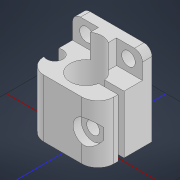
# Autodesk Inventor part: Vinda_Mount_v2
Saved by Autodesk Inventor 2022 (Build 260153000, 153)
## iProperties
Created: 2022-02-14
Part Number: Vinda_Mount_v2
Material: Stahl
Document SubType Name: Modeling
Designer: sleib
Density: 7.85 g/cm^3
Appearance: Vorgabe
Sending System: Autodesk Translation Framework v10.10.0.1391
Preprocessor: ST-DEVELOPER v18.1
Title: C:/Users/sleib/Projekte/Voron-2/STLs/VORON2.4/Gantry/X_Axis/X_Carriage/Vinda_Mount v4.step
Autodesk Inventor part; units mm, degrees
ref_plane "YZ Plane" through (0, 0, 0) normal (1, 0, 0) x (0, 1, 0)
ref_plane "XZ Plane" through (0, 0, 0) normal (0, 1, 0) x (-1, 0, 0)
ref_plane "XY Plane" through (0, 0, 0) normal (0, 0, 1) x (1, 0, 0)
sketch "Skizze2" plane through (0, 0, 0) normal (0, 1, 0) x (-1, 0, 0)
  arc A0 (-3.9291, -0.75) -> (-3.9291, 0.75) centre (0, 0) ccw
  line L0 (8.75, -7.7556) -> (-8.75, -7.7556)
  line L1 (-8.75, -7.7556) -> (-8.75, 5.8)
  line L2 (-8.75, 5.8) -> (8.75, 5.8)
  line L3 (8.75, 5.8) -> (8.75, -7.7556)
  line L4 (8.75, -4.6225) -> (8.75, -1.5) projected
  arc A1 (8.75, 1.8) -> (8.75, -1.8) centre (7.8242, 0) ccw
  line L5 (8.75, -7.7556) -> (-8.75, -7.7556)
  line L6 (-8.75, -7.7556) -> (-8.75, -5.3556)
  line L7 (-8.75, -5.3556) -> (8.75, -5.3556)
  line L8 (8.75, -5.3556) -> (8.75, -7.7556)
  line L9 (2.25, -5.3556) -> (2.25, -3.3072)
  line L10 (-2.25, -5.3556) -> (-2.25, -3.3072)
  arc A2 (-2.25, -3.3072) -> (2.25, -3.3072) centre (0, 0) ccw
  line L11 (2.25, -5.3556) -> (-2.25, -5.3556)
  line L12 (-3.9291, -0.75) -> (-8.75, -0.75)
  line L13 (-3.9291, 0.75) -> (-8.75, 0.75)
  arc A3 (8.75, 1.8) -> (4.75, 5.8) centre (4.75, 1.8) ccw
  arc A4 (-4.75, 5.8) -> (-8.75, 1.8) centre (-4.75, 1.8) ccw
  line L14 (0, -10.6323) -> (0, 9.5052) construction
  line L15 (8.75, 0) -> (-8.75, 0) construction
  point P0 (5.25, -5.3556)
  point P1 (-5.25, -5.3556)
  dimension "d0" = 8
  dimension "d2" = 17.5
  dimension "d4" = 1.8
  dimension "d7" = 2.4
  dimension "d8" = 1.5
  dimension "d10" = 4
  dimension "d11" = 10.5
  dimension "d12" = 3
  dimension "d38" = 1.8
  dimension "d39" = 1.3556
  constraints: 30 end point, 16 point on line, 12 point on circle, 5 centre point, 5 perpendicular, 4 parallel, 4 tangent, 3 collinear, 3 horizontal, 2 equal radius, 2 midpoint, 1 symmetric about line, 3 other
  measures "d0" diameter of A0
  measures "d2" distance of L0.start L0.end
  measures "d7" distance between parallel lines of L7 L5
  measures "d8" distance between parallel lines of L13 L12
  measures "d10" radius of A3
  measures "d11" distance of point (-5.25, -5.356) point (5.25, -5.356)
  measures "d12" distance from line of L9 point (5.25, -5.356)
  measures "d38" distance edge to line of A0 L2
  measures "d39" distance edge to line of A0 L11
extrude "Extrusion2" add sketch "Skizze2" against normal blind 14.5 contours A0 L10 L7 L1 L12 | A0 L9 L7 L10 | A0 L13 L1 A4 L2 A3 A1 L3 L7 L9 | L7 L3 L0 L1
extrude "Extrusion3" add sketch "Skizze2" along normal blind 6 contours A0 L9 L7 L10 | L7 L3 L0 L1
sketch "Skizze3" plane through (-8.75, 0, -5.3556) normal (0, 0, 1) x (1, 0, 0)
  line L0 (0, -14.5) -> (0, 0) projected
  line L1 (0, 0) -> (0, 6) projected
  line L2 (0, 6) -> (6.5, 6) projected
  line L3 (6.5, 6) -> (11, 6) projected
  line L4 (11, 6) -> (11, 0) projected
  line L5 (11, 0) -> (17.5, 0) projected
  line L6 (17.5, 6) -> (17.5, 0) projected
  line L7 (11, 6) -> (17.5, 6) projected
  line L8 (17.5, -14.5) -> (0, -14.5) projected
  line L9 (17.5, 0) -> (17.5, -14.5) projected
  line L10 (0, 0) -> (6.5, 0) projected
  line L11 (6.5, 0) -> (6.5, 6) projected
  line L12 (3.5, 0) -> (3.5, 6) construction
  line L13 (0, 6) -> (6.5, 6) projected
  line L14 (14, 0) -> (14, 6) construction
  line L15 (11, 6) -> (17.5, 6) projected
  point P0 (8.75, 0)
  point P1 (3.5, 3)
  point P2 (14, 3)
  constraints: 4 end point, 2 midpoint, 2 perpendicular, 2 point on line
hole "Bohrung1" at (-5.25, 3, -5.3556) at (5.25, 3, -5.3556) direction (0, 0, -1) diameter 3.4 end through all clearance for "Inbusschraube DIN EN ISO 4762" size "M3" standard "DIN"
fillet "Rundung1" radius 2 2 edges at (-8.75, 6, -6.5556) (8.75, 6, -6.5556)
sketch "Skizze4" plane through (-4.75, 0, 5.8) normal (0, 0, 1) x (1, 0, 0)
  line L0 (8.6791, 0) -> (13.5, 0) projected
  line L1 (8.6791, 0) -> (8.6791, -14.5) projected
  line L2 (13.5, -14.5) -> (8.6791, -14.5) projected
  line L3 (13.5, 0) -> (13.5, -14.5) projected
  line L4 (13.5, 0) -> (9.5, 0) projected
  line L5 (10.3, -14.5) -> (10.3, 0) construction
  point P0 (4.75, 0)
  point P1 (10.3, -7.25)
  dimension "d30" = 3.2
  constraints: 2 end point, 2 point on line, 1 midpoint, 1 vertical
  measures "d30" distance between parallel lines of L3 L5
hole "Bohrung2" at (5.55, -7.25, 5.8) direction (0, 0, -1) diameter 3.2 end through all counterbore diameter 6 counterbore depth 2 clearance for "Inbusschraube DIN EN ISO 4762" size "M3" standard "DIN"
sketch "Skizze5" plane through (8.75, -14.5, -7.7556) normal (0, 0, -1) x (-1, 0, 0)
  circle A0 centre (3.2, 7.25) radius 1.6 projected
  point P0 (8.75, 14.5)
hole "Bohrung3" at (5.55, -7.25, -7.7556) direction (0, 0, 1) diameter 4.5 depth 5
